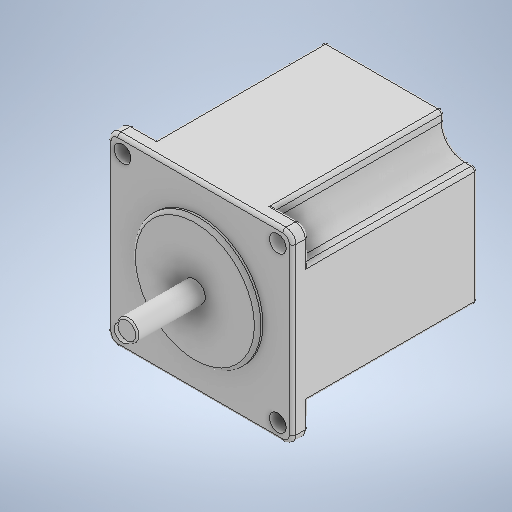
# Autodesk Inventor part: silnik_krokowy_W56.4xH56.4xL56
Saved by Autodesk Inventor 2025.2 (Build 292293000, 293)
## iProperties
Created: 2025-03-19
Part Number: silnik_krokowy_W56.4xH56.4xL56
Material: Ogólny
Document SubType Name: Modeling
Designer: rango
Density: 1 g/cm^3
Appearance: Domyślna
Author: rango
Autodesk Inventor part; units mm, degrees
ref_plane "YZ Plane" through (0, 0, 0) normal (1, 0, 0) x (0, 1, 0)
ref_plane "XZ Plane" through (0, 0, 0) normal (0, 1, 0) x (-1, 0, 0)
ref_plane "XY Plane" through (0, 0, 0) normal (0, 0, 1) x (1, 0, 0)
sketch "Szkic1" plane through (0, 0, 0) normal (0, 0, 1) x (1, 0, 0)
  line L0 (28, 28) -> (-28, 28)
  line L1 (-28, 28) -> (-28, -28)
  line L2 (-28, -28) -> (28, -28)
  line L3 (28, -28) -> (28, 28)
  line L4 (-18, 28) -> (-18, 25)
  line L5 (-28, 18) -> (-25, 18)
  line L6 (-18, -28) -> (-18, -25)
  line L7 (-28, -18) -> (-25, -18)
  line L8 (28, -18) -> (25, -18)
  line L9 (28, 18) -> (25, 18)
  line L10 (18, 28) -> (18, 25)
  arc A0 (-25, 18) -> (-18, 25) centre (-25, 25) ccw
  arc A1 (18, 25) -> (25, 18) centre (25, 25) ccw
  arc A2 (-18, -25) -> (-25, -18) centre (-25, -25) ccw
  line L11 (18, -28) -> (18, -25)
  arc A3 (25, -18) -> (18, -25) centre (25, -25) ccw
  point P0 (0, 0)
  dimension "d0" = 56
  dimension "d1" = 56
  dimension "d2" = 3
  dimension "d3" = 3
  dimension "d4" = 3
  dimension "d5" = 3
  dimension "d6" = 3
  dimension "d7" = 3
  dimension "d8" = 3
  dimension "d9" = 3
  constraints: 24 end point, 8 point on circle, 8 point on line, 8 tangent, 5 perpendicular, 4 centre point, 3 vertical, 2 horizontal, 2 parallel
  measures "d0" distance of L2.end L1.end
  measures "d1" distance of L1.end L0.end
  measures "d2" distance of L4.start L4.end
  measures "d3" distance of L5.start L5.end
  measures "d4" distance of L6.start L6.end
  measures "d5" distance of L7.start L7.end
  measures "d6" distance of L8.start L8.end
  measures "d7" distance of L9.start L9.end
  measures "d8" distance of L10.start L10.end
  measures "d9" distance of L11.start L11.end
extrude "Wyciągnięcie proste1" add sketch "Szkic1" along normal blind 51.2 contours L10 A1 L9 L3 L8 A3 L11 L2 L6 A2 L7 L1 L5 A0 L4 L0
sketch "Szkic2" plane through (0, 0, 51.2) normal (0, 0, 1) x (1, 0, 0)
  line L0 (-28, 28) -> (28, 28)
  line L1 (28, 28) -> (28, -28)
  line L2 (28, -28) -> (-28, -28)
  line L3 (-28, -28) -> (-28, 28)
  point P0 (0, 0)
  dimension "d12" = 56
  constraints: 8 end point, 2 parallel, 1 horizontal, 1 perpendicular
  measures "d12" distance of L0.end L1.end
extrude "Wyciągnięcie proste2" add sketch "Szkic2" along normal blind 4.8
fillet "Zaokrąglenie1" radius 3 4 edges at (28, 28, 53.6) (-28, 28, 53.6) (28, -28, 53.6) (-28, -28, 53.6)
sketch "Szkic3" plane through (0, 0, 56) normal (0, 0, 1) x (1, 0, 0)
  line L0 (-23.5, 28) -> (-23.5, 23.5)
  circle A0 centre (-23.5, 23.5) radius 2.55
  circle A1 centre (23.5, 23.5) radius 2.55
  circle A2 centre (23.5, -23.5) radius 2.55
  circle A3 centre (-23.5, -23.5) radius 2.55
  point P0 (0, 0)
  dimension "d16" = 4.5
  dimension "d17" = 5.1
  dimension "d18" = 5.1
  dimension "d19" = 5.1
  dimension "d20" = 5.1
  constraints: 4 centre point, 2 end point, 1 coincident, 1 vertical
  measures "d16" distance of L0.start L0.end
  measures "d17" diameter of A0
  measures "d18" diameter of A1
  measures "d19" diameter of A2
  measures "d20" diameter of A3
extrude "Wyciągnięcie proste3" cut sketch "Szkic3" against normal blind 4.8
fillet "Zaokrąglenie2" radius 1 44 edges at (18, 28, 25.6) (28, 18, 25.6) (28, -18, 25.6) (18, -28, 25.6) (-18, -28, 25.6) (-28, -18, 25.6) (-28, 18, 25.6) (-18, 28, 25.6) (-27.1213, 27.1213, 56) (-28, 0, 56) (-27.1213, -27.1213, 56) (0, -28, 56) (27.1213, -27.1213, 56) (28, 0, 56) (27.1213, 27.1213, 56) (0, 28, 56) (-27.1213, 27.1213, 51.2) (-21.5, 28, 51.2) (-28, 21.5, 51.2) (-27.1213, -27.1213, 51.2) (-21.5, -28, 51.2) (-28, -21.5, 51.2) (27.1213, -27.1213, 51.2) (28, -21.5, 51.2) (21.5, -28, 51.2) (27.1213, 27.1213, 51.2) (21.5, 28, 51.2) (28, 21.5, 51.2) (26.5, -18, 0) (18, -26.5, 0) (20.0503, -20.0503, 0) (0, -28, 0) (28, 0, 0) (18, 26.5, 0) (26.5, 18, 0) (20.0503, 20.0503, 0) (0, 28, 0) (-26.5, 18, 0) (-18, 26.5, 0) (-20.0503, 20.0503, 0) (-28, 0, 0) (-18, -26.5, 0) (-26.5, -18, 0) (-20.0503, -20.0503, 0)
sketch "Szkic4" plane through (0, 0, 56) normal (0, 0, 1) x (1, 0, 0)
  circle A0 centre (0, 0) radius 19
  dimension "d24" = 38
  constraints: 1 centre point, 1 coincident
  measures "d24" diameter of A0
extrude "Wyciągnięcie proste4" add sketch "Szkic4" along normal blind 1.6
fillet "Zaokrąglenie3" radius 1 1 edges at (-19, 0, 57.6)
sketch "Szkic5" plane through (0, 0, 57.6) normal (0, 0, 1) x (1, 0, 0)
  circle A0 centre (0, 0) radius 3.18
  dimension "d28" = 6.36
  constraints: 1 centre point, 1 coincident
  measures "d28" diameter of A0
extrude "Wyciągnięcie proste5" add sketch "Szkic5" along normal blind 20.6
fillet "Zaokrąglenie4" radius 0.5 1 edges at (-3.18, 0, 78.2)
